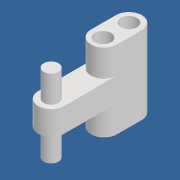
# Autodesk Inventor part: Crank0
Saved by Autodesk Inventor 2020 (Build 240168000, 168)
## iProperties
Created: 2019-12-22
Part Number: Crank0
Material: Generic
Document SubType Name: Modeling
Designer: Jack
Density: 1 g/cm^3
Appearance: Default
Author: Jack
Autodesk Inventor part; units mm, degrees
ref_plane "YZ Plane" through (0, 0, 0) normal (1, 0, 0) x (0, 1, 0)
ref_plane "XZ Plane" through (0, 0, 0) normal (0, 1, 0) x (-1, 0, 0)
ref_plane "XY Plane" through (0, 0, 0) normal (0, 0, 1) x (1, 0, 0)
sketch "Sketch1" plane through (0, 0, 0) normal (0, 1, 0) x (-1, 0, 0)
  line L0 (0, 0) -> (-8, 0)
  line L1 (-8, 0) -> (-8, -15.7)
  line L2 (-8, -15.7) -> (0, -15.7)
  line L3 (0, -15.7) -> (0, 0)
  circle A0 centre (-4, -3.7) radius 2.5
  circle A1 centre (-4, -11.7) radius 2.5
  dimension "d0" = 8
  dimension "d1" = 15.7
  dimension "d4" = 5
  dimension "d5" = 5
  dimension "d8" = 8
  dimension "d15" = 4
  constraints: 8 end point, 2 centre point, 2 parallel, 1 horizontal, 1 perpendicular, 1 vertical alignment
  measures "d0" distance of L2.end L1.end
  measures "d1" distance of L1.end L0.end
  measures "d4" diameter of A0
  measures "d5" diameter of A1
  measures "d8" distance of A1.centre A0.centre
  measures "d15" distance from line of L1 A1.centre
extrude "Extrusion1" add sketch "Sketch1" along normal blind 24
fillet "Fillet1" radius 4 2 edges at (8, 12, 0) (0, 12, 0)
fillet "Fillet2" radius 4 2 edges at (8, 12, -15.7) (0, 12, -15.7)
sketch "Sketch2" plane through (0, 0, -4) normal (-1, 0, 0) x (0, 0, 1)
  line L0 (0, 8.3) -> (20.3, 8.3)
  line L1 (20.3, 8.3) -> (20.3, 15.7)
  line L2 (20.3, 15.7) -> (0, 15.7)
  line L3 (0, 15.7) -> (0, 8.3)
  line L4 (0, 24) -> (4, 24) projected
  line L5 (0, 24) -> (0, 0) projected
  point P0 (4, 0)
  dimension "d17" = 20.3
  dimension "d18" = 7.4
  dimension "d19" = 8.3
  constraints: 8 end point, 2 parallel, 1 horizontal, 1 perpendicular, 1 point on line
  measures "d17" distance of L2.end L1.end
  measures "d18" distance of L1.end L0.end
  measures "d19" distance between parallel lines of L4 L2
extrude "Extrusion2" add sketch "Sketch2" against normal blind 8
sketch "Sketch4" plane through (0, 15.7, 16.3) normal (0, 1, 0) x (1, 0, 0)
  circle A0 centre (4, 4) radius 2.3
  line L0 (8, 20.3) -> (8, 0) projected
  line L1 (0, 0) -> (8, 0) projected
  point P0 (0, 16.3)
  point P1 (8, 12)
  dimension "d24" = 4.6
  dimension "d25" = 4
  dimension "d26" = 4
  constraints: 1 centre point
  measures "d24" diameter of A0
  measures "d25" distance from line of L0 A0.centre
  measures "d26" distance from line of L1 A0.centre
extrude "Extrusion4" add sketch "Sketch4" along normal blind 8.3 and the other way blind 15.7
fillet "Fillet3" radius 4 2 edges at (0, 12, 16.3) (8, 12, 16.3)
body "Solid1"
